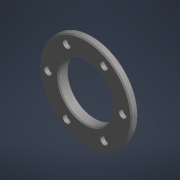
# Autodesk Inventor part: SeguroRodamientos
Saved by Autodesk Inventor 2022 (Build 260153000, 153)
## iProperties
Created: 2021-09-21
Part Number: SeguroRodamientos
Material: Steel, Mild, Welded
Document SubType Name: Modeling
Designer: Andres
Density: 7.85 g/cm^3
Appearance: Weld - Steel Mild
Author: Andres
Autodesk Inventor part; units mm, degrees
ref_plane "YZ Plane" through (0, 0, 0) normal (1, 0, 0) x (0, 1, 0)
ref_plane "XZ Plane" through (0, 0, 0) normal (0, 1, 0) x (-1, 0, 0)
ref_plane "XY Plane" through (0, 0, 0) normal (0, 0, 1) x (1, 0, 0)
sketch "Sketch1" plane through (0, 0, 0) normal (0, 0, 1) x (1, 0, 0)
  circle A0 centre (0, 0) radius 40 projected
  circle A1 centre (0, 0) radius 28 projected
  circle A2 centre (0, 0) radius 23.5
  circle A3 centre (-16.25, -28.1458) radius 1.621 projected
  circle A4 centre (-16.25, 28.1458) radius 1.621 projected
  circle A5 centre (32.5, 0) radius 1.621 projected
  circle A6 centre (16.25, 28.1458) radius 1.621 projected
  circle A7 centre (-32.5, 0) radius 1.621 projected
  circle A8 centre (16.25, -28.1458) radius 1.621 projected
  dimension "d0" = 47
  constraints: 1 centre point, 1 coincident
  measures "d0" diameter of A2
ref_plane "Work Plane3" through (-60, -60, 6) normal (0, 0, 1) x (1, 0, 0)
extrude "Extrusion3" add sketch "Sketch1" along normal up to surface (6 mm away) contours A0 | A1 | A3 | A4 | A5 | A6 | A7 | A8
sketch "Sketch4" plane through (0, 0, 0) normal (0, 0, -1) x (-1, 0, 0)
  circle A0 centre (0, 0) radius 23.5 projected
  circle A1 centre (0, 0) radius 26 projected
ref_plane "Work Plane4" through (-29.7534, -29.7534, -2) normal (0, 0, 1) x (0.9818774, -0.1895171, 0)
extrude "Extrusion4" add sketch "Sketch4" along normal up to surface (2 mm away)
chamfer "Chamfer4" distance 2 angle 45 1 edges at (26, 0, 0)
chamfer "Chamfer5" distance 1 angle 45 2 edges at (-40, 0, 6) (-23.5, 0, 6)
sketch "Sketch5" plane through (0, 0, 6) normal (0, 0, 1) x (1, 0, 0)
  circle A0 centre (0, 0) radius 32.5 construction
  point P0 (32.5, 0)
  point P1 (16.25, 28.1458)
  point P2 (-16.25, 28.1458)
  point P3 (-32.5, 0)
  point P4 (-16.25, -28.1458)
  point P5 (16.25, -28.1458)
  dimension "d36" = 65
  dimension "d39" = 360
  constraints: 2 horizontal alignment, 1 coincident, 9 other
hole "Hole2" at (32.5, 0, 6) at (16.25, 28.1458, 6) at (-16.25, 28.1458, 6) at (-32.5, 0, 6) at (-16.25, -28.1458, 6) at (16.25, -28.1458, 6) direction (0, 0, -1) diameter 3.4 end through all counterbore diameter 6.5 counterbore depth 3.4 clearance for "Socket Head Cap Screw ISO 4762" size "M3" standard "ISO"
chamfer "Chamfer6" distance 1 angle 45 1 edges at (-40, 0, 0)
body "Solid2"
